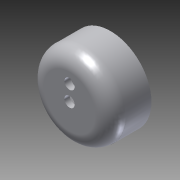
# Autodesk Inventor part: Motor End Cap
Saved by Autodesk Inventor 2013 (Build 170138000, 138)
## iProperties
Created: 2013-07-29
Part Number: Motor End Cap
Material: PVC-Piping
Document SubType Name: Modeling
Designer: Kyle
Density: 1 g/cm^3
Author: Kyle
Autodesk Inventor part; units mm, degrees
ref_plane "YZ Plane" through (0, 0, 0) normal (1, 0, 0) x (0, 1, 0)
sketch "Sketch1" plane through (0, 0, 0) normal (0, 0, 1) x (1, 0, 0)
  circle A0 centre (0, 0) radius 16.51
  circle A1 centre (0, 0) radius 20.32
  dimension "d0" = 40.64
  dimension "d2" = 33.02
  constraints: 2 centre point, 1 coincident
  measures "d0" diameter of A1
  measures "d2" diameter of A0
extrude "Extrusion1" add sketch "Sketch1" along normal blind 11.43
sketch "Sketch2" plane through (0, 0, 11.43) normal (0, 0, 1) x (1, 0, 0)
  circle A0 centre (0, 0) radius 20.32 projected
  circle A1 centre (0, 0) radius 15.875
  dimension "d5" = 31.75
  constraints: 1 centre point, 1 coincident
  measures "d5" diameter of A1
extrude "Extrusion2" add sketch "Sketch2" along normal blind 1.27
fillet "Fillet1" radius 0.508 1 edges at (-15.875, 0, 11.43)
fillet "Fillet2" radius 0.508 1 edges at (-15.875, 0, 12.7)
ref_plane "Work Plane1" through (0, 0, 6.35) normal (0, 0, 1) x (1, 0, 0)
sketch "Sketch3" plane through (0, 0, 6.35) normal (0, 0, 1) x (1, 0, 0)
  line L0 (-20.32, 19.1494) -> (-20.32, -22.3588)
  circle A0 centre (0, 0) radius 20.32 projected
  dimension "d11" = 20.32
  constraints: 2 end point, 1 vertical
  measures "d11" distance from line of L0 A0.centre
sketch "Sketch4" plane through (0, 0, 12.7) normal (0, 0, 1) x (1, 0, 0)
  circle A0 centre (0, 0) radius 20.32 projected
  circle A1 centre (0, 0) radius 16.383 projected
ref_plane "Work Plane3" through (-20.32, 19.1494, 6.35) normal (-1, 0, 0) x (0, -1, 0)
ref_plane "Work Plane2" through (0, 0, 12.7) normal (0, 0, 1) x (1, 0, 0)
ref_plane "Work Plane4" through (0, 19.1494, 6.35) normal (-1, 0, 0) x (0, -1, 0)
sketch "Sketch6" plane through (0, 19.1494, 6.35) normal (-1, 0, 0) x (0, -1, 0)
  line L0 (39.364, 6.35) -> (35.554, 6.35)
  arc A0 (35.554, 6.35) -> (20.314, 11.4045) centre (19.0928, -17.78) ccw
  line L1 (39.364, 6.35) -> (39.364, 6.35)
  line L2 (31.744, 13.97) -> (20.314, 13.97)
  line L3 (20.314, 13.97) -> (20.314, 11.4045)
  arc A1 (39.364, 6.35) -> (31.744, 13.97) centre (31.744, 6.35) ccw
  line L4 (39.4694, 6.35) -> (-1.1706, 6.35) projected
  line L5 (19.044, 13.97) -> (19.044, 8.477)
  point P0 (19.1494, -6.35)
  point P1 (19.044, 5.9584)
  point P2 (19.044, 27.5056)
  point P3 (19.044, 11.43)
  point P4 (39.364, 13.97)
  dimension "d24" = 3.81
  dimension "d25" = 20.32
  dimension "d26" = 5.08
  dimension "d27" = 29.21
  dimension "d28" = 7.62
  dimension "d29" = 7.62
  dimension "d30" = 0
  constraints: 10 end point, 4 point on circle, 3 perpendicular, 2 centre point, 2 point on line, 2 tangent, 1 horizontal
  measures "d24" distance of L0.start L0.end
  measures "d25" horizontal distance of point (19.044, 5.958) L0.start
  measures "d26" distance from line of point (19.044, 11.43) L0
  measures "d27" radius of A0
  measures "d28" distance of L0.start point (39.364, 13.97)
  measures "d29" radius of A1
  measures "d30" distance between parallel lines of L4 L0
revolve "Revolution1" add sketch "Sketch6" angle 360 about axis through (0, 0.1054, 20.32) along (0, 0, -1)
sketch "Sketch7" plane through (0, 0.1054, 20.32) normal (0, 0, 1) x (1, 0, 0)
  circle A0 centre (0, 0) radius 1.27 projected
  point P0 (0, -0.1054)
extrude "Extrusion3" add sketch "Sketch7" against normal blind 2.5654
sketch "Sketch8" plane through (0, 0.1054, 20.32) normal (0, 0, 1) x (1, 0, 0)
  circle A0 centre (0, 0) radius 12.7 projected
  circle A1 centre (0, 0) radius 2.54
  circle A2 centre (0, 7.6441) radius 2.54
  point P0 (0, -0.1054)
  dimension "d34" = 5.08
  dimension "d36" = 5.08
  constraints: 2 centre point, 1 coincident
  measures "d34" diameter of A1
  measures "d36" diameter of A2
extrude "Extrusion4" cut sketch "Sketch8" against normal blind 25.4 contours A1 | A2
body "Solid1"
